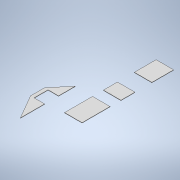
# Autodesk Inventor part: 零件1
Saved by Autodesk Inventor 2021 (Build 250183000, 183)
## iProperties
Created: 2022-10-06
Part Number: 零件1
Material: 一般
Document SubType Name: Modeling
Designer: 生活科技
Density: 1 g/cm^3
Appearance: 預設
Author: 生活科技
Autodesk Inventor part; units mm, degrees
ref_plane "YZ Plane" through (0, 0, 0) normal (1, 0, 0) x (0, 1, 0)
ref_plane "XZ Plane" through (0, 0, 0) normal (0, 1, 0) x (-1, 0, 0)
ref_plane "XY Plane" through (0, 0, 0) normal (0, 0, 1) x (1, 0, 0)
sketch "草圖1" plane through (0, 0, 0) normal (0, 1, 0) x (-1, 0, 0)
  line L0 (104.3168, 198.8324) -> (-195.6832, 198.8324)
  line L1 (204.3168, 198.8324) -> (-195.6832, 891.6528)
  line L2 (-195.6832, 891.6528) -> (-195.6832, 198.8324)
  line L3 (204.3168, 198.8324) -> (204.3168, -201.1676)
  line L4 (104.3168, -201.1676) -> (-195.6832, -201.1676)
  line L5 (204.3168, -201.1676) -> (-195.6832, -677.869)
  line L6 (-195.6832, -201.1676) -> (-195.6832, -677.869)
  line L7 (104.3168, 198.8324) -> (104.3168, -201.1676)
  line L8 (-696.9674, 126.681) -> (-1196.9674, 126.681)
  line L9 (-1196.9674, 126.681) -> (-1196.9674, -673.319)
  line L10 (-1196.9674, -673.319) -> (-696.9674, -673.319)
  line L11 (-696.9674, -673.319) -> (-696.9674, 126.681)
  line L12 (-696.9674, 126.681) -> (-1196.9674, -673.319) construction
  line L13 (-1196.9674, 126.681) -> (-696.9674, -673.319) construction
  line L14 (-1196.9674, -1385.819) -> (-696.9674, -1385.819)
  line L15 (-696.9674, -1385.819) -> (-696.9674, -985.819)
  line L16 (-696.9674, -985.819) -> (-1196.9674, -985.819)
  line L17 (-1196.9674, -985.819) -> (-1196.9674, -1385.819)
  line L18 (-1196.9674, -1385.819) -> (-696.9674, -985.819) construction
  line L19 (-696.9674, -1385.819) -> (-1196.9674, -985.819) construction
  line L20 (-1196.9674, -2493.949) -> (-696.9674, -2493.949)
  line L21 (-696.9674, -2493.949) -> (-696.9674, -1871.659)
  line L22 (-696.9674, -1871.659) -> (-1196.9674, -1871.659)
  line L23 (-1196.9674, -1871.659) -> (-1196.9674, -2493.949)
  line L24 (-1196.9674, -2493.949) -> (-696.9674, -1871.659) construction
  line L25 (-696.9674, -2493.949) -> (-1196.9674, -1871.659) construction
  point P0 (-946.9674, -273.319)
  point P1 (-946.9674, -1185.819)
  point P2 (-946.9674, -2182.804)
  dimension "d3" = 30
  dimension "d6" = 400
  dimension "d8" = 400
  dimension "d10" = 100
  dimension "d11" = 40
  dimension "d12" = 800
  dimension "d13" = 622.2895
  dimension "d18" = 800
  dimension "d19" = 500
  dimension "d20" = 400
  dimension "d21" = 500
  dimension "d22" = 622.29
  dimension "d23" = 500
  constraints: 52 end point, 6 midpoint, 6 parallel, 5 horizontal, 4 perpendicular, 3 vertical
  measures "d3" angle of L2 L1
  measures "d6" distance of L1.start L0.end
  measures "d8" distance of L1.start L3.end
  measures "d10" distance between parallel lines of L7 L3
  measures "d11" angle of L6 L5
  measures "d12" distance of L1.start L1.end
  measures "d13" distance of L3.end L5.end
  measures "d18" distance of L10.end L8.start
  measures "d19" distance of L9.end L10.end
  measures "d20" distance of L14.end L15.end
  measures "d21" distance of L14.start L14.end
  measures "d22" distance of L20.end L21.end
  measures "d23" distance of L20.start L20.end
extrude "擠出1" add sketch "草圖1" along normal blind 10
